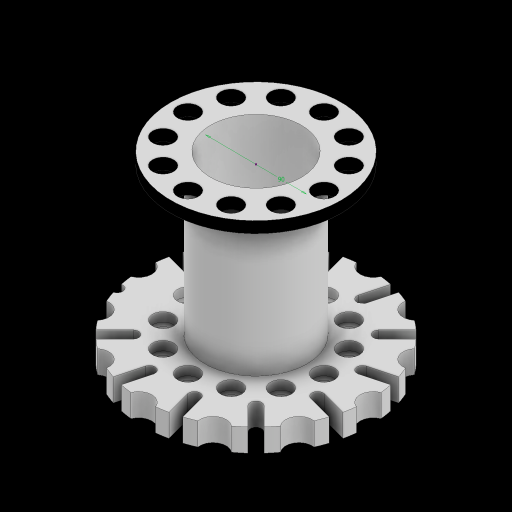
# Autodesk Inventor part: 12 Test Tube Rack
Saved by Autodesk Inventor 2023 (Build 270158000, 158)
## iProperties
Created: 2022-10-22
Part Number: 12 Test Tube Rack
Material: Generic
Document SubType Name: Modeling
Designer: annah
Density: 1 g/cm^3
Appearance: Default
Author: annah
Autodesk Inventor part; units mm, degrees
ref_plane "YZ Plane" through (0, 0, 0) normal (1, 0, 0) x (0, 1, 0)
ref_plane "XZ Plane" through (0, 0, 0) normal (0, 1, 0) x (-1, 0, 0)
ref_plane "XY Plane" through (0, 0, 0) normal (0, 0, 1) x (1, 0, 0)
sketch "Sketch1" plane through (0, 0, 0) normal (0, 1, 0) x (-1, 0, 0)
  circle A0 centre (0, 0) radius 75
  circle A1 centre (0, 0) radius 60
  circle A2 centre (0, 60) radius 9.25
  circle A3 centre (-30, 51.9615) radius 9.25
  circle A4 centre (-51.9615, 30) radius 9.25
  circle A5 centre (-60, 0) radius 9.25
  circle A6 centre (-51.9615, -30) radius 9.25
  circle A7 centre (-30, -51.9615) radius 9.25
  circle A8 centre (0, -60) radius 9.25
  circle A9 centre (30, -51.9615) radius 9.25
  circle A10 centre (51.9615, -30) radius 9.25
  circle A11 centre (60, 0) radius 9.25
  circle A12 centre (51.9615, 30) radius 9.25
  circle A13 centre (30, 51.9615) radius 9.25
  dimension "d1" = 120
  dimension "d0" = 150
  dimension "d2" = 18.5
  dimension "d5" = 360
  constraints: 13 centre point, 2 coincident, 1 vertical alignment, 27 other
  measures "d0" diameter of A0
  measures "d2" diameter of A2
extrude "Extrusion1" add sketch "Sketch1" along normal blind 10 contours A0 | A11 A1 A10 A9 A8 A7 A6 A5 A4 A3 A2 A13 A12
sketch "Sketch2" plane through (0, 0, 0) normal (0, -1, 0) x (1, 0, 0)
  circle A0 centre (0, 0) radius 45
  dimension "d9" = 90
  constraints: 1 centre point, 1 coincident
  measures "d9" diameter of A0
extrude "Extrusion2" add sketch "Sketch2" along normal blind 130
sketch "Sketch3" plane through (0, -130, 0) normal (0, -1, 0) x (1, 0, 0)
  circle A0 centre (0, 0) radius 5
  line L0 (-11.0031, 74.0969) -> (11.0031, 74.0969)
  line L1 (11.0031, 74.0969) -> (11.0031, 56.269)
  line L2 (11.0031, 56.269) -> (-11.0031, 56.269)
  line L3 (-11.0031, 56.269) -> (-11.0031, 74.0969)
  line L4 (11.0031, 74.0969) -> (0, 65.183) construction
  line L5 (-27.5195, 69.6713) -> (-18.6056, 54.232)
  line L6 (-18.6056, 54.232) -> (-37.6635, 43.2289)
  line L7 (-37.6635, 43.2289) -> (-46.5774, 58.6682)
  line L8 (-46.5774, 58.6682) -> (-27.5195, 69.6713)
  line L9 (-58.6682, 46.5774) -> (-43.2289, 37.6635)
  line L10 (-43.2289, 37.6635) -> (-54.232, 18.6056)
  line L11 (-54.232, 18.6056) -> (-69.6713, 27.5195)
  line L12 (-69.6713, 27.5195) -> (-58.6682, 46.5774)
  line L13 (-74.0969, 11.0031) -> (-56.269, 11.0031)
  line L14 (-56.269, 11.0031) -> (-56.269, -11.0031)
  line L15 (-56.269, -11.0031) -> (-74.0969, -11.0031)
  line L16 (-74.0969, -11.0031) -> (-74.0969, 11.0031)
  line L17 (-69.6713, -27.5195) -> (-54.232, -18.6056)
  line L18 (-54.232, -18.6056) -> (-43.2289, -37.6635)
  line L19 (-43.2289, -37.6635) -> (-58.6682, -46.5774)
  line L20 (-58.6682, -46.5774) -> (-69.6713, -27.5195)
  line L21 (-46.5774, -58.6682) -> (-37.6635, -43.2289)
  line L22 (-37.6635, -43.2289) -> (-18.6056, -54.232)
  line L23 (-18.6056, -54.232) -> (-27.5195, -69.6713)
  line L24 (-27.5195, -69.6713) -> (-46.5774, -58.6682)
  line L25 (-11.0031, -74.0969) -> (-11.0031, -56.269)
  line L26 (-11.0031, -56.269) -> (11.0031, -56.269)
  line L27 (11.0031, -56.269) -> (11.0031, -74.0969)
  line L28 (11.0031, -74.0969) -> (-11.0031, -74.0969)
  line L29 (27.5195, -69.6713) -> (18.6056, -54.232)
  line L30 (18.6056, -54.232) -> (37.6635, -43.2289)
  line L31 (37.6635, -43.2289) -> (46.5774, -58.6682)
  line L32 (46.5774, -58.6682) -> (27.5195, -69.6713)
  line L33 (58.6682, -46.5774) -> (43.2289, -37.6635)
  line L34 (43.2289, -37.6635) -> (54.232, -18.6056)
  line L35 (54.232, -18.6056) -> (69.6713, -27.5195)
  line L36 (69.6713, -27.5195) -> (58.6682, -46.5774)
  line L37 (74.0969, -11.0031) -> (56.269, -11.0031)
  line L38 (56.269, -11.0031) -> (56.269, 11.0031)
  line L39 (56.269, 11.0031) -> (74.0969, 11.0031)
  line L40 (74.0969, 11.0031) -> (74.0969, -11.0031)
  line L41 (69.6713, 27.5195) -> (54.232, 18.6056)
  line L42 (54.232, 18.6056) -> (43.2289, 37.6635)
  line L43 (43.2289, 37.6635) -> (58.6682, 46.5774)
  line L44 (58.6682, 46.5774) -> (69.6713, 27.5195)
  line L45 (46.5774, 58.6682) -> (37.6635, 43.2289)
  line L46 (37.6635, 43.2289) -> (18.6056, 54.232)
  line L47 (18.6056, 54.232) -> (27.5195, 69.6713)
  line L48 (27.5195, 69.6713) -> (46.5774, 58.6682)
  arc A1 (-11.0031, 60.9667) -> (-20.9544, 58.3003) centre (0, 0) ccw
  arc A2 (20.9544, 58.3003) -> (11.0031, 60.9667) centre (0, 0) ccw
  arc A3 (47.2972, 40.0123) -> (40.0123, 47.2972) centre (0, 0) ccw
  arc A4 (-40.0123, 47.2972) -> (-47.2972, 40.0123) centre (0, 0) ccw
  arc A5 (-58.3003, 20.9544) -> (-60.9667, 11.0031) centre (0, 0) ccw
  arc A6 (-60.9667, -11.0031) -> (-58.3003, -20.9544) centre (0, 0) ccw
  arc A7 (-47.2972, -40.0123) -> (-40.0123, -47.2972) centre (0, 0) ccw
  arc A8 (-20.9544, -58.3003) -> (-11.0031, -60.9667) centre (0, 0) ccw
  arc A9 (11.0031, -60.9667) -> (20.9544, -58.3003) centre (0, 0) ccw
  arc A10 (40.0123, -47.2972) -> (47.2972, -40.0123) centre (0, 0) ccw
  arc A11 (58.3003, -20.9544) -> (60.9667, -11.0031) centre (0, 0) ccw
  arc A12 (60.9667, 11.0031) -> (58.3003, 20.9544) centre (0, 0) ccw
  dimension "d68" = 360
  constraints: 98 end point, 24 point on circle, 24 point on line, 13 centre point, 3 coincident, 2 parallel, 1 horizontal, 1 perpendicular, 97 other
extrude "Extrusion9" add sketch "Sketch3" along normal blind 10
sketch "Sketch7" plane through (0, -130, 0) normal (0, 1, 0) x (1, 0, 0)
  circle A0 centre (0, 0) radius 5 projected
  circle A1 centre (0, 0) radius 60
  circle A2 centre (-60, 0) radius 9.25
  circle A3 centre (-51.9615, -30) radius 9.25
  circle A4 centre (-30, -51.9615) radius 9.25
  circle A5 centre (0, -60) radius 9.25
  circle A6 centre (30, -51.9615) radius 9.25
  circle A7 centre (51.9615, -30) radius 9.25
  circle A8 centre (60, 0) radius 9.25
  circle A9 centre (51.9615, 30) radius 9.25
  circle A10 centre (30, 51.9615) radius 9.25
  circle A11 centre (0, 60) radius 9.25
  circle A12 centre (-30, 51.9615) radius 9.25
  circle A13 centre (-51.9615, 30) radius 9.25
  dimension "d71" = 120
  dimension "d72" = 18.5
  dimension "d75" = 360
  constraints: 12 centre point, 1 coincident, 1 horizontal alignment, 27 other
  measures "d72" diameter of A2
extrude "Extrusion10" cut sketch "Sketch7" against normal blind 10 contours A1 A8 | A1 A8 | A9 A1 | A1 A9 | A7 A1 | A1 A7 | A10 A1 | A1 A10 | A6 A1 | A1 A6 | A11 A1 | A1 A11 | A5 A1 | A1 A5 | A12 A1 | A1 A12 | A4 A1 | A1 A4 | A13 A1 | A1 A13 | A3 A1 | A1 A3 | A2 A1 | A1 A2
sketch "Sketch8" plane through (0, 10, 0) normal (0, 1, 0) x (1, 0, 0)
  circle A0 centre (0, 0) radius 5 projected
  circle A1 centre (0, 0) radius 40
  dimension "d92" = 80
  constraints: 1 centre point, 1 coincident
  measures "d92" diameter of A1
extrude "Extrusion11" cut sketch "Sketch8" against normal blind 140 contours A0 | A1
sketch "Sketch9" plane through (0, -140, 0) normal (0, -1, 0) x (1, 0, 0)
  circle A0 centre (0, 0) radius 100
  line L0 (0, 0) -> (18.5658, -69.2885)
  line L1 (0, 0) -> (0, -103.5276)
  arc A1 (24.6448, -72.6673) -> (14.9907, -75.2542) centre (0, 0) ccw
  circle A2 centre (25.8819, -96.5926) radius 5
  arc A3 (24.729, -72.9816) -> (15.0747, -75.5678) centre (19.8599, -74.1181) ccw
  line L2 (30.6777, -95.1782) -> (24.6448, -72.6673)
  line L3 (21.0523, -97.8867) -> (14.9907, -75.2542)
  circle A4 centre (0, -103.5276) radius 11.6229
  line L4 (21.0523, -97.8867) -> (25.8819, -96.5926)
  arc A5 (-25.8819, -96.5926) -> (26.7197, -101.5219) centre (0, -103.5276) ccw
  circle A6 centre (0, -103.5276) radius 40
  arc A7 (57.9067, -50.8394) -> (50.8389, -57.9063) centre (54.2582, -54.2582) ccw
  line L5 (67.1751, -74.2462) -> (50.6094, -57.6767)
  line L6 (74.1567, -67.0879) -> (57.6767, -50.6094)
  circle A8 centre (70.7107, -70.7107) radius 5
  circle A9 centre (51.7638, -89.6575) radius 11.6229
  arc A10 (75.5684, -15.0748) -> (72.9809, -24.7289) centre (74.1181, -19.8599) ccw
  line L7 (95.2985, -30.7115) -> (72.6673, -24.6448)
  line L8 (97.7655, -21.0214) -> (75.2542, -14.9907)
  circle A11 centre (96.5926, -25.8819) radius 5
  circle A12 centre (89.6575, -51.7638) radius 11.6229
  arc A13 (72.9816, 24.729) -> (75.5678, 15.0747) centre (74.1181, 19.8599) ccw
  line L9 (97.8867, 21.0523) -> (75.2542, 14.9907)
  line L10 (95.1782, 30.6777) -> (72.6673, 24.6448)
  circle A14 centre (96.5926, 25.8819) radius 5
  circle A15 centre (103.5276, 0) radius 11.6229
  arc A16 (50.8394, 57.9067) -> (57.9063, 50.8389) centre (54.2582, 54.2582) ccw
  line L11 (74.2462, 67.1751) -> (57.6767, 50.6094)
  line L12 (67.0879, 74.1567) -> (50.6094, 57.6767)
  circle A17 centre (70.7107, 70.7107) radius 5
  circle A18 centre (89.6575, 51.7638) radius 11.6229
  arc A19 (15.0748, 75.5684) -> (24.7289, 72.9809) centre (19.8599, 74.1181) ccw
  line L13 (30.7115, 95.2985) -> (24.6448, 72.6673)
  line L14 (21.0214, 97.7655) -> (14.9907, 75.2542)
  circle A20 centre (25.8819, 96.5926) radius 5
  circle A21 centre (51.7638, 89.6575) radius 11.6229
  arc A22 (-24.729, 72.9816) -> (-15.0747, 75.5678) centre (-19.8599, 74.1181) ccw
  line L15 (-21.0523, 97.8867) -> (-14.9907, 75.2542)
  line L16 (-30.6777, 95.1782) -> (-24.6448, 72.6673)
  circle A23 centre (-25.8819, 96.5926) radius 5
  circle A24 centre (0, 103.5276) radius 11.6229
  arc A25 (-57.9067, 50.8394) -> (-50.8389, 57.9063) centre (-54.2582, 54.2582) ccw
  line L17 (-67.1751, 74.2462) -> (-50.6094, 57.6767)
  line L18 (-74.1567, 67.0879) -> (-57.6767, 50.6094)
  circle A26 centre (-70.7107, 70.7107) radius 5
  circle A27 centre (-51.7638, 89.6575) radius 11.6229
  arc A28 (-75.5684, 15.0748) -> (-72.9809, 24.7289) centre (-74.1181, 19.8599) ccw
  line L19 (-95.2985, 30.7115) -> (-72.6673, 24.6448)
  line L20 (-97.7655, 21.0214) -> (-75.2542, 14.9907)
  circle A29 centre (-96.5926, 25.8819) radius 5
  circle A30 centre (-89.6575, 51.7638) radius 11.6229
  arc A31 (-72.9816, -24.729) -> (-75.5678, -15.0747) centre (-74.1181, -19.8599) ccw
  line L21 (-97.8867, -21.0523) -> (-75.2542, -14.9907)
  line L22 (-95.1782, -30.6777) -> (-72.6673, -24.6448)
  circle A32 centre (-96.5926, -25.8819) radius 5
  circle A33 centre (-103.5276, 0) radius 11.6229
  arc A34 (-50.8394, -57.9067) -> (-57.9063, -50.8389) centre (-54.2582, -54.2582) ccw
  line L23 (-74.2462, -67.1751) -> (-57.6767, -50.6094)
  line L24 (-67.0879, -74.1567) -> (-50.6094, -57.6767)
  circle A35 centre (-70.7107, -70.7107) radius 5
  circle A36 centre (-89.6575, -51.7638) radius 11.6229
  arc A37 (-15.0748, -75.5684) -> (-24.7289, -72.9809) centre (-19.8599, -74.1181) ccw
  line L25 (-30.7115, -95.2985) -> (-24.6448, -72.6673)
  line L26 (-21.0214, -97.7655) -> (-14.9907, -75.2542)
  circle A38 centre (-25.8819, -96.5926) radius 5
  circle A39 centre (-51.7638, -89.6575) radius 11.6229
  circle A40 centre (0, 0) radius 3
  circle A41 centre (0, -103.5276) radius 2.5
  point P0 (50.7227, -50.7227)
  point P1 (73.9009, -74.5607)
  point P2 (69.2885, -18.5658)
  point P3 (101.2804, -27.621)
  point P4 (69.2885, 18.5658)
  point P5 (101.5219, 26.7197)
  point P6 (50.7227, 50.7227)
  point P7 (74.5607, 73.9009)
  point P8 (18.5658, 69.2885)
  point P9 (27.621, 101.2804)
  point P10 (-18.5658, 69.2885)
  point P11 (-26.7197, 101.5219)
  point P12 (-50.7227, 50.7227)
  point P13 (-73.9009, 74.5607)
  point P14 (-69.2885, 18.5658)
  point P15 (-101.2804, 27.621)
  point P16 (-69.2885, -18.5658)
  point P17 (-101.5219, -26.7197)
  point P18 (-50.7227, -50.7227)
  point P19 (-74.5607, -73.9009)
  point P20 (-18.5658, -69.2885)
  point P21 (-27.621, -101.2804)
  point P22 (40.2917, -91.5236)
  point P23 (59.1159, -80.6555)
  point P24 (67.0867, -74.1578)
  point P25 (80.6555, -59.1159)
  point P26 (91.5236, -40.2917)
  point P27 (95.1777, -30.6791)
  point P28 (99.4077, -10.8682)
  point P29 (99.4077, 10.8682)
  point P30 (97.7659, 21.0199)
  point P31 (91.5236, 40.2917)
  point P32 (80.6555, 59.1159)
  point P33 (74.1578, 67.0867)
  point P34 (59.1159, 80.6555)
  point P35 (40.2917, 91.5236)
  point P36 (30.6791, 95.1777)
  point P37 (10.8682, 99.4077)
  point P38 (-10.8682, 99.4077)
  point P39 (-21.0199, 97.7659)
  point P40 (-40.2917, 91.5236)
  point P41 (-59.1159, 80.6555)
  point P42 (-67.0867, 74.1578)
  point P43 (-80.6555, 59.1159)
  point P44 (-91.5236, 40.2917)
  point P45 (-95.1777, 30.6791)
  point P46 (-99.4077, 10.8682)
  point P47 (-99.4077, -10.8682)
  point P48 (-97.7659, -21.0199)
  point P49 (-91.5236, -40.2917)
  point P50 (-80.6555, -59.1159)
  point P51 (-74.1578, -67.0867)
  point P52 (-59.1159, -80.6555)
  point P53 (-40.2917, -91.5236)
  point P54 (-30.6791, -95.1777)
  point P55 (-10.8682, -99.4077)
  point P56 (10.8682, -99.4077)
  point P57 (21.0199, -97.7659)
  point P58 (20.4557, -69.1537)
  point P59 (24.2422, -71.7107)
  point P60 (40.2917, -91.5236)
  point P61 (59.1159, -80.6555)
  point P62 (67.0867, -74.1578)
  point P63 (80.6555, -59.1159)
  point P64 (91.5236, -40.2917)
  point P65 (95.1777, -30.6791)
  point P66 (99.4077, -10.8682)
  point P67 (99.4077, 10.8682)
  point P68 (97.7659, 21.0199)
  point P69 (91.5236, 40.2917)
  point P70 (80.6555, 59.1159)
  point P71 (74.1578, 67.0867)
  point P72 (59.1159, 80.6555)
  point P73 (40.2917, 91.5236)
  point P74 (30.6791, 95.1777)
  point P75 (10.8682, 99.4077)
  point P76 (-10.8682, 99.4077)
  point P77 (-21.0199, 97.7659)
  point P78 (-40.2917, 91.5236)
  point P79 (-59.1159, 80.6555)
  point P80 (-67.0867, 74.1578)
  point P81 (-80.6555, 59.1159)
  point P82 (-91.5236, 40.2917)
  point P83 (-95.1782, 30.6777)
  point P84 (-99.4077, 10.8682)
  point P85 (-99.4077, -10.8682)
  point P86 (-97.7659, -21.0199)
  point P87 (-91.5236, -40.2917)
  point P88 (-80.6555, -59.1159)
  point P89 (-74.1578, -67.0867)
  point P90 (-59.1159, -80.6555)
  point P91 (-40.2917, -91.5236)
  point P92 (-30.6791, -95.1777)
  point P93 (-24.2422, -71.7107)
  point P94 (-20.4557, -69.1537)
  point P95 (-10.8682, -99.4077)
  point P96 (10.8682, -99.4077)
  point P97 (21.0199, -97.7659)
  dimension "d97" = 200
  dimension "d98" = 15
  dimension "d99" = 10
  dimension "d100" = 10
  dimension "d101" = 80
  dimension "d102" = 360
  dimension "d103" = 6
  dimension "d104" = 5
  constraints: 100 point on circle, 54 end point, 41 centre point, 25 point on line, 8 coincident, 1 vertical, 198 other
  measures "d98" angle of L1 L0
  measures "d99" diameter of A2
  measures "d100" diameter of A3
  measures "d101" diameter of A6
  measures "d103" diameter of A40
  measures "d104" diameter of A41
extrude "Extrusion12" add sketch "Sketch9" along normal blind 10 contours L26 A37 A1 L1 A4 A0 | A0 A6 A1 A37 L25 | A0 A39 L24 A34 A1 A6 | L1 A1 A3 L3 A0 A4 | A37 A6 L1 A1 | A6 A37 A1 | A1 A34 A31 A28 A25 A22 A19 A16 A13 A10 A7 A6 A3 L0 A40 L1 A37 | L1 A6 L0 A3 A1 | A6 A37 | A6 A1 A7 L5 A0 A9 | A0 L2 A3 A1 A6 | L1 A40 L0 A6 | A34 L23 A0 A36 L22 A31 A1 | A1 A3 A6 | A40 L0 L1 | L1 L0 A40 | A6 A3 L0 | A6 A3 | A31 L21 A0 A33 L20 A28 A1 | A1 A10 L7 A0 A12 L6 A7 | A28 L20 A29 L19 A1 | A1 A28 | A28 L19 A0 A30 L18 A25 A1 | A1 A13 L9 A0 A15 L8 A10 | A25 L17 A0 A27 L16 A22 A1 | A1 A16 L11 A0 A18 L10 A13 | A22 L15 A0 A24 L14 A19 A1 | A1 A19 L13 A0 A21 L12 A16 picked at (-24.7526, -72.3861)
sketch "Sketch10" plane through (0, -140, 0) normal (0, 1, 0) x (1, 0, 0)
  arc A0 (20.4557, 69.1537) -> (24.2422, 71.7107) centre (0, 103.5276) ccw projected
  arc A1 (14.9907, 75.2542) -> (20.4557, 69.1537) centre (19.8599, 74.1181) ccw projected
  line L0 (21.0199, 97.7659) -> (14.9907, 75.2542) projected
  arc A2 (21.0199, 97.7659) -> (10.8682, 99.4077) centre (0, 0) ccw projected
  arc A3 (-10.8682, 99.4077) -> (10.8682, 99.4077) centre (0, 103.5276) ccw projected
  arc A4 (-10.8682, 99.4077) -> (-21.0214, 97.7655) centre (0, 0) ccw projected
  line L1 (-14.9907, 75.2542) -> (-21.0214, 97.7655) projected
  arc A5 (-20.4557, 69.1537) -> (-14.9907, 75.2542) centre (-19.8599, 74.1181) ccw projected
  arc A6 (-24.2422, 71.7107) -> (-20.4557, 69.1537) centre (0, 103.5276) ccw projected
  arc A7 (-24.6448, 72.6673) -> (-24.2422, 71.7107) centre (-19.8599, 74.1181) ccw projected
  line L2 (-30.6791, 95.1777) -> (-24.6448, 72.6673) projected
  arc A8 (-30.6791, 95.1777) -> (-40.2917, 91.5236) centre (0, 0) ccw projected
  arc A9 (-59.1159, 80.6555) -> (-40.2917, 91.5236) centre (-51.7638, 89.6575) ccw projected
  arc A10 (-59.1159, 80.6555) -> (-67.0879, 74.1567) centre (0, 0) ccw projected
  line L3 (-50.6094, 57.6767) -> (-67.0879, 74.1567) projected
  arc A11 (-57.6767, 50.6094) -> (-50.6094, 57.6767) centre (-54.2582, 54.2582) ccw projected
  line L4 (-74.1578, 67.0867) -> (-57.6767, 50.6094) projected
  arc A12 (-74.1578, 67.0867) -> (-80.6555, 59.1159) centre (0, 0) ccw projected
  arc A13 (-91.5236, 40.2917) -> (-80.6555, 59.1159) centre (-89.6575, 51.7638) ccw projected
  arc A14 (-91.5236, 40.2917) -> (-95.1782, 30.6777) centre (0, 0) ccw projected
  line L5 (-72.6673, 24.6448) -> (-95.1782, 30.6777) projected
  arc A15 (-75.2542, 14.9907) -> (-72.6673, 24.6448) centre (-74.1181, 19.8599) ccw projected
  line L6 (-97.7659, 21.0199) -> (-75.2542, 14.9907) projected
  arc A16 (-97.7659, 21.0199) -> (-99.4077, 10.8682) centre (0, 0) ccw projected
  arc A17 (-99.4077, -10.8682) -> (-99.4077, 10.8682) centre (-103.5276, 0) ccw projected
  arc A18 (-99.4077, -10.8682) -> (-97.7655, -21.0214) centre (0, 0) ccw projected
  arc A19 (-95.1782, -30.6777) -> (-97.7655, -21.0214) centre (-96.5926, -25.8819) ccw projected
  arc A20 (-95.1782, -30.6777) -> (-91.5236, -40.2917) centre (0, 0) ccw projected
  arc A21 (-80.6555, -59.1159) -> (-91.5236, -40.2917) centre (-89.6575, -51.7638) ccw projected
  arc A22 (-80.6555, -59.1159) -> (-74.1567, -67.0879) centre (0, 0) ccw projected
  line L7 (-57.6767, -50.6094) -> (-74.1567, -67.0879) projected
  arc A23 (-50.6094, -57.6767) -> (-57.6767, -50.6094) centre (-54.2582, -54.2582) ccw projected
  line L8 (-67.0867, -74.1578) -> (-50.6094, -57.6767) projected
  arc A24 (-67.0867, -74.1578) -> (-59.1159, -80.6555) centre (0, 0) ccw projected
  arc A25 (-40.2917, -91.5236) -> (-59.1159, -80.6555) centre (-51.7638, -89.6575) ccw projected
  arc A26 (-40.2917, -91.5236) -> (-30.6777, -95.1782) centre (0, 0) ccw projected
  line L9 (-24.6448, -72.6673) -> (-30.6777, -95.1782) projected
  arc A27 (-14.9907, -75.2542) -> (-24.6448, -72.6673) centre (-19.8599, -74.1181) ccw projected
  line L10 (-21.0199, -97.7659) -> (-14.9907, -75.2542) projected
  arc A28 (-21.0199, -97.7659) -> (-10.8682, -99.4077) centre (0, 0) ccw projected
  arc A29 (10.8682, -99.4077) -> (-10.8682, -99.4077) centre (0, -103.5276) ccw projected
  arc A30 (10.8682, -99.4077) -> (21.0214, -97.7655) centre (0, 0) ccw projected
  line L11 (14.9907, -75.2542) -> (21.0214, -97.7655) projected
  arc A31 (24.6448, -72.6673) -> (14.9907, -75.2542) centre (19.8599, -74.1181) ccw projected
  line L12 (30.6791, -95.1777) -> (24.6448, -72.6673) projected
  arc A32 (30.6791, -95.1777) -> (40.2917, -91.5236) centre (0, 0) ccw projected
  arc A33 (59.1159, -80.6555) -> (40.2917, -91.5236) centre (51.7638, -89.6575) ccw projected
  arc A34 (59.1159, -80.6555) -> (67.0879, -74.1567) centre (0, 0) ccw projected
  line L13 (50.6094, -57.6767) -> (67.0879, -74.1567) projected
  arc A35 (57.6767, -50.6094) -> (50.6094, -57.6767) centre (54.2582, -54.2582) ccw projected
  line L14 (74.1578, -67.0867) -> (57.6767, -50.6094) projected
  arc A36 (74.1578, -67.0867) -> (80.6555, -59.1159) centre (0, 0) ccw projected
  arc A37 (91.5236, -40.2917) -> (80.6555, -59.1159) centre (89.6575, -51.7638) ccw projected
  arc A38 (91.5236, -40.2917) -> (95.1782, -30.6777) centre (0, 0) ccw projected
  line L15 (72.6673, -24.6448) -> (95.1782, -30.6777) projected
  arc A39 (75.2542, -14.9907) -> (72.6673, -24.6448) centre (74.1181, -19.8599) ccw projected
  line L16 (97.7659, -21.0199) -> (75.2542, -14.9907) projected
  arc A40 (97.7659, -21.0199) -> (99.4077, -10.8682) centre (0, 0) ccw projected
  arc A41 (99.4077, 10.8682) -> (99.4077, -10.8682) centre (103.5276, 0) ccw projected
  arc A42 (99.4077, 10.8682) -> (97.7655, 21.0214) centre (0, 0) ccw projected
  line L17 (75.2542, 14.9907) -> (97.7655, 21.0214) projected
  arc A43 (72.6673, 24.6448) -> (75.2542, 14.9907) centre (74.1181, 19.8599) ccw projected
  line L18 (95.1777, 30.6791) -> (72.6673, 24.6448) projected
  arc A44 (95.1777, 30.6791) -> (91.5236, 40.2917) centre (0, 0) ccw projected
  arc A45 (80.6555, 59.1159) -> (91.5236, 40.2917) centre (89.6575, 51.7638) ccw projected
  arc A46 (80.6555, 59.1159) -> (74.1567, 67.0879) centre (0, 0) ccw projected
  line L19 (57.6767, 50.6094) -> (74.1567, 67.0879) projected
  arc A47 (50.6094, 57.6767) -> (57.6767, 50.6094) centre (54.2582, 54.2582) ccw projected
  line L20 (67.0867, 74.1578) -> (50.6094, 57.6767) projected
  arc A48 (67.0867, 74.1578) -> (59.1159, 80.6555) centre (0, 0) ccw projected
  arc A49 (40.2917, 91.5236) -> (59.1159, 80.6555) centre (51.7638, 89.6575) ccw projected
  arc A50 (40.2917, 91.5236) -> (30.6777, 95.1782) centre (0, 0) ccw projected
  line L21 (24.6448, 72.6673) -> (30.6777, 95.1782) projected
  arc A51 (24.2422, 71.7107) -> (24.6448, 72.6673) centre (19.8599, 74.1181) ccw projected
  line L22 (60.9667, 11.0031) -> (74.0969, 11.0031) projected
  line L23 (74.0969, 11.0031) -> (74.0969, -11.0031) projected
  line L24 (74.0969, -11.0031) -> (60.9667, -11.0031) projected
  arc A52 (58.3003, -20.9544) -> (60.9667, -11.0031) centre (0, 0) ccw projected
  line L25 (58.3003, -20.9544) -> (69.6713, -27.5195) projected
  line L26 (69.6713, -27.5195) -> (58.6682, -46.5774) projected
  line L27 (58.6682, -46.5774) -> (47.2972, -40.0123) projected
  arc A53 (40.0123, -47.2972) -> (47.2972, -40.0123) centre (0, 0) ccw projected
  line L28 (40.0123, -47.2972) -> (46.5774, -58.6682) projected
  line L29 (46.5774, -58.6682) -> (27.5195, -69.6713) projected
  line L30 (27.5195, -69.6713) -> (20.9544, -58.3003) projected
  arc A54 (11.0031, -60.9667) -> (20.9544, -58.3003) centre (0, 0) ccw projected
  line L31 (11.0031, -60.9667) -> (11.0031, -74.0969) projected
  line L32 (11.0031, -74.0969) -> (-11.0031, -74.0969) projected
  line L33 (-11.0031, -74.0969) -> (-11.0031, -60.9667) projected
  arc A55 (-20.9544, -58.3003) -> (-11.0031, -60.9667) centre (0, 0) ccw projected
  line L34 (-20.9544, -58.3003) -> (-27.5195, -69.6713) projected
  line L35 (-27.5195, -69.6713) -> (-46.5774, -58.6682) projected
  line L36 (-46.5774, -58.6682) -> (-40.0123, -47.2972) projected
  arc A56 (-47.2972, -40.0123) -> (-40.0123, -47.2972) centre (0, 0) ccw projected
  line L37 (-47.2972, -40.0123) -> (-58.6682, -46.5774) projected
  line L38 (-58.6682, -46.5774) -> (-69.6713, -27.5195) projected
  line L39 (-69.6713, -27.5195) -> (-58.3003, -20.9544) projected
  arc A57 (-60.9667, -11.0031) -> (-58.3003, -20.9544) centre (0, 0) ccw projected
  line L40 (-60.9667, -11.0031) -> (-74.0969, -11.0031) projected
  line L41 (-74.0969, -11.0031) -> (-74.0969, 11.0031) projected
  line L42 (-74.0969, 11.0031) -> (-60.9667, 11.0031) projected
  arc A58 (-58.3003, 20.9544) -> (-60.9667, 11.0031) centre (0, 0) ccw projected
  line L43 (-58.3003, 20.9544) -> (-69.6713, 27.5195) projected
  line L44 (-69.6713, 27.5195) -> (-58.6682, 46.5774) projected
  line L45 (-58.6682, 46.5774) -> (-47.2972, 40.0123) projected
  arc A59 (-40.0123, 47.2972) -> (-47.2972, 40.0123) centre (0, 0) ccw projected
  line L46 (-40.0123, 47.2972) -> (-46.5774, 58.6682) projected
  line L47 (-46.5774, 58.6682) -> (-27.5195, 69.6713) projected
  line L48 (-27.5195, 69.6713) -> (-20.9544, 58.3003) projected
  arc A60 (-11.0031, 60.9667) -> (-20.9544, 58.3003) centre (0, 0) ccw projected
  line L49 (-11.0031, 60.9667) -> (-11.0031, 74.0969) projected
  line L50 (-11.0031, 74.0969) -> (11.0031, 74.0969) projected
  line L51 (11.0031, 74.0969) -> (11.0031, 60.9667) projected
  arc A61 (20.9544, 58.3003) -> (11.0031, 60.9667) centre (0, 0) ccw projected
  line L52 (20.9544, 58.3003) -> (27.5195, 69.6713) projected
  line L53 (27.5195, 69.6713) -> (46.5774, 58.6682) projected
  line L54 (46.5774, 58.6682) -> (40.0123, 47.2972) projected
  arc A62 (47.2972, 40.0123) -> (40.0123, 47.2972) centre (0, 0) ccw projected
  line L55 (47.2972, 40.0123) -> (58.6682, 46.5774) projected
  line L56 (58.6682, 46.5774) -> (69.6713, 27.5195) projected
  line L57 (69.6713, 27.5195) -> (58.3003, 20.9544) projected
  arc A63 (60.9667, 11.0031) -> (58.3003, 20.9544) centre (0, 0) ccw projected
extrude "Extrusion13" add sketch "Sketch10" along normal blind 10
fillet "Fillet2" radius 2 12 edges at (20.75, -140, 51.9615) (42.7115, -140, 30) (50.75, -140, 0) (42.7115, -140, -30) (20.75, -140, -51.9615) (-9.25, -140, -60) (-39.25, -140, -51.9615) (-9.25, -140, 60) (-39.25, -140, 51.9615) (-61.2115, -140, 30) (-69.25, -140, 0) (-61.2115, -140, -30)
body "Solid1"
